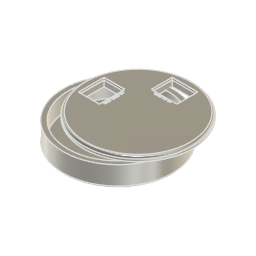
sEMG_sensorCasing (Autodesk Fusion 360 design; units mm, degrees)
Autodesk Fusion 360 part; units mm, degrees
cylinder "CylinderPrimitive1" add diameter 43 height 7 placed x (1, 0, 0) y (0, 1, 0) z (0, 0, 1) at (0, 0, 0) makes body 1
shell "Shell1" thickness 2 outward yes removed faces 1 at (-0.08, 1.0681, 7) on bodies 1
sketch "Sketch2" plane through (0, 0, 7) normal (0, 0, 1) x (-1, 0, 0)
  circle A0 centre (0, 0) radius 21.5
  circle A1 centre (0, 0) radius 23.5
  circle A2 centre (0, 0) radius 21.5
  circle A3 centre (0, 0) radius 23.5
  circle A4 centre (0, 0) radius 21.68
  dimension "d8" = 0.18
extrude "Extrude1" add sketch "Sketch2" along normal blind 2 separate body contours A0 A2 | A1 A3 | A4 makes body 2
extrude "Extrude2" add sketch "Sketch2" against normal blind 1 contours A0 A2 bodies 2
sketch "Sketch3" plane through (0, 0, 9) normal (0, 0, 1) x (-1, 0, 0)
  circle A0 centre (0, 0) radius 23.5
  circle A1 centre (0, 0) radius 21.68
  line L0 (19.68, -5) -> (11.68, -5)
  line L1 (11.68, -5) -> (11.68, 5)
  line L2 (11.68, 5) -> (19.68, 5)
  line L3 (19.68, 5) -> (19.68, -5)
  line L4 (19.68, 0) -> (11.68, 0) construction
  line L5 (21.68, 4) -> (21.68, -4) construction
  line L6 (-5, -19.68) -> (-5, -11.68)
  line L7 (-5, -11.68) -> (5, -11.68)
  line L8 (5, -11.68) -> (5, -19.68)
  line L9 (5, -19.68) -> (-5, -19.68)
  point P0 (21.68, 0)
  point P1 (21.68, 0)
  dimension "d15" = 8
  dimension "d16" = 10
  dimension "d17" = 2
  dimension "d18" = 2
  dimension "d19" = 2
  dimension "d21" = 270
  constraint horizontal L0
  constraint vertical L1
  constraint horizontal L2
  constraint vertical L3
  constraint midpoint L3 L4.start
  constraint midpoint L1 L4.end
  constraint coincident L4 A0.centre
  constraint coincident A1 P1
  constraint vertical L5
  constraint tangent A1 L5
  measures "d15" distance of L0.start L0.end
  measures "d16" distance of L0.end L1.end
  measures "d17" horizontal distance of L4.start P1
  measures "d18" distance of L3 P1
  measures "d19" distance of L3 L5
extrude "Extrude3" cut sketch "Sketch3" against normal through all contours L0 L1 L2 L3 | L6 L7 L8 L9 bodies 2
sketch "Sketch4" plane through (0, 0, 9) normal (0, 0, 1) x (-1, 0, 0)
  line L0 (19.68, 5) -> (19.68, -5)
  line L1 (19.68, -5) -> (11.68, -5)
  line L2 (11.68, -5) -> (11.68, 5)
  line L3 (11.68, 5) -> (19.68, 5)
  line L4 (5, -19.68) -> (-5, -19.68)
  line L5 (-5, -19.68) -> (-5, -11.68)
  line L6 (-5, -11.68) -> (5, -11.68)
  line L7 (5, -11.68) -> (5, -19.68)
  circle A0 centre (0, 0) radius 23.5
  line L8 (9.793, 4.9526) -> (9.793, -4.9785) construction
  line L9 (9.793, -4.9785) -> (11.1756, -4.9785) construction
  line L10 (11.1756, -4.9785) -> (11.1756, 4.9526) construction
  line L11 (11.1756, 4.9526) -> (9.793, 4.9526) construction
  line L12 (5.0173, -9.9822) -> (-5.0141, -9.9822) construction
  line L13 (-5.0141, -9.9822) -> (-5.0141, -11.3039) construction
  line L14 (-5.0141, -11.3039) -> (5.0173, -11.3039) construction
  line L15 (5.0173, -11.3039) -> (5.0173, -9.9822) construction
  dimension "d23" = 1
  dimension "d24" = 1
  text T0 "OUT GND V+" font "Arial" height 1 align centre middle in box 9.9311 x 1.3826 at (9.793, 4.9526) x (0, -1) y (1, 0) spacing 1 kerned
  text T1 "GND V+ V-" font "Arial" height 1 align centre middle in box 10.0314 x 1.3217 at (5.0173, -9.9822) x (-1, 0) y (0, -1) spacing 1 kerned
extrude "Extrude4" cut sketch "Sketch4" against normal blind 0.5 text T0 T1 bodies 2
fillet "Fillet1" radius 1 2 edges at (-21.9097, 8.498, -2) (21.9097, 8.498, 9) on bodies 1 2
fillet "Fillet2" radius 0.5 8 edges at (-19.68, 0, 9) (-15.68, 5, 9) (-15.68, -5, 9) (-11.68, 0, 9) (-5, 15.68, 9) (0, 19.68, 9) (0, 11.68, 9) (5, 15.68, 9) on bodies 2
copy_body "Body->Comp1" bodies 2 removing the originals makes body 3 in component "Component"
component "Component" placed x (1, 0, 0) y (0, 1, 0) z (0, 0, 1) at (0, 0, 0)
equation "diametro = 43 mm"
equation "alto = 7 mm"
equation "Grosor = 2 mm"
equation "tolerancia = 0.18 mm"
equation "d5 = alto"
equation "d6 = diametro"
equation "d7 = Grosor"
equation "d8 = tolerancia"
equation "d9 = Grosor"
equation "d11 = -Grosor / 2"
equation "ancho = 8 mm"
equation "largoPin = 10 mm"
equation "d15 = ancho"
equation "d16 = largoPin"
equation "redondeo = 1 mm"
equation "d29 = redondeo"
equation "d31 = redondeo / 2"
